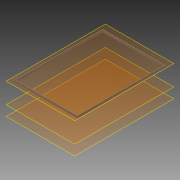
# Autodesk Inventor part: Basic Frame
Saved by Autodesk Inventor 2015 (Build 190159000, 159)
## iProperties
Created: 2016-01-18
Part Number: Basic Frame
Material: Generic
Document SubType Name: Modeling
Designer: sethbattis
Density: 1 g/cm^3
Appearance: Default
Author: sethbattis
Autodesk Inventor part; units mm, degrees
ref_plane "YZ Plane" through (0, 0, 0) normal (1, 0, 0) x (0, 1, 0)
ref_plane "XY Plane" through (0, 0, 0) normal (0, 0, 1) x (1, 0, 0)
ref_plane "Ground Plane" through (0, -220.9292, 0) normal (0, 1, 0) x (-1, 0, 0)
ref_plane "Lower Bumper Plane" through (0, -119.3292, 0) normal (0, 1, 0) x (-1, 0, 0)
ref_plane "Upper Bumper Plane" through (0, 83.8708, 0) normal (0, 1, 0) x (-1, 0, 0)
sketch "Sketch5" plane through (0, 83.8708, 0) normal (0, 1, 0) x (-1, 0, 0)
  line L0 (435.61, 0) -> (-435.61, 0) projected
  line L1 (0, -613.41) -> (0, 613.41) projected
  line L2 (311.15, -438.15) -> (-311.15, -438.15)
  line L3 (-311.15, -438.15) -> (-311.15, 438.15)
  line L4 (-311.15, 438.15) -> (311.15, 438.15)
  line L5 (311.15, 438.15) -> (311.15, -438.15)
  line L6 (307.975, -434.975) -> (-307.975, -434.975)
  line L7 (-307.975, -434.975) -> (-307.975, 434.975)
  line L8 (-307.975, 434.975) -> (307.975, 434.975)
  line L9 (307.975, 434.975) -> (307.975, -434.975)
  point P0 (0, 0)
  dimension "d29" = 622.3
  dimension "d30" = 876.3
  dimension "d31" = 3.175
  dimension "d32" = 3.175
  dimension "d33" = 3.175
  dimension "d34" = 3.175
  constraints: 16 end point, 4 parallel, 2 horizontal, 2 perpendicular, 2 other
  measures "d29" distance of L3.end L4.end
  measures "d30" distance of L2.end L3.end
  measures "d31" distance between parallel lines of L2 L6
  measures "d32" distance between parallel lines of L4 L8
  measures "d33" distance between parallel lines of L3 L7
  measures "d34" distance between parallel lines of L5 L9
extrude "Extrusion6" add sketch "Sketch5" against normal blind 25.4 contours L5 L2 L1 L6 L9 L0 | L0 L9 L8 L1 L4 L5 | L1 L8 L7 L0 L3 L4 | L2 L3 L0 L7 L6 L1
body "Solid3"
